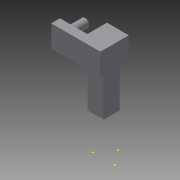
# Autodesk Inventor part: BearingEndCap
Saved by Autodesk Inventor 2015 (Build 190159000, 159)
## iProperties
Created: 2016-03-24
Part Number: BearingEndCap
Material: Generic
Document SubType Name: Modeling
Designer: Hatch
Density: 1 g/cm^3
Appearance: Default
Author: Hatch
Autodesk Inventor part; units mm, degrees
ref_plane "YZ Plane" through (0, 0, 0) normal (1, 0, 0) x (0, 1, 0)
ref_plane "XZ Plane" through (0, 0, 0) normal (0, 1, 0) x (-1, 0, 0)
ref_plane "XY Plane" through (0, 0, 0) normal (0, 0, 1) x (1, 0, 0)
sketch "Sketch1" plane through (0, 0, 0) normal (0, 1, 0) x (-1, 0, 0)
  line L0 (-7.25, 7.25) -> (7.25, 7.25)
  line L1 (7.25, 7.25) -> (7.25, -7.25)
  line L2 (7.25, -7.25) -> (-7.25, -7.25)
  line L3 (-7.25, -7.25) -> (-7.25, 7.25)
  line L4 (-7.25, 7.25) -> (7.25, -7.25) construction
  line L5 (7.25, 7.25) -> (-7.25, -7.25) construction
  point P0 (0, 0)
  dimension "d0" = 14.5
  dimension "d1" = 14.5
  constraints: 12 end point, 2 midpoint, 2 parallel, 1 horizontal, 1 perpendicular
  measures "d0" distance of L1.end L2.end
  measures "d1" distance of L0.end L1.end
extrude "Extrusion1" add sketch "Sketch1" along normal blind 76.2
sketch "Sketch2" plane through (0, 76.2, 0) normal (0, 1, 0) x (1, 0, 0)
  line L0 (10, -10) -> (-10, -10)
  line L1 (-10, -10) -> (-10, 10)
  line L2 (-10, 10) -> (10, 10)
  line L3 (10, 10) -> (10, -10)
  line L4 (10, -10) -> (-10, 10) construction
  line L5 (-10, -10) -> (10, 10) construction
  point P0 (0, 0)
  dimension "d4" = 20
  dimension "d5" = 20
  constraints: 12 end point, 2 midpoint, 2 parallel, 1 horizontal, 1 perpendicular
  measures "d4" distance of L1.end L2.end
  measures "d5" distance of L0.end L1.end
extrude "Extrusion2" add sketch "Sketch2" along normal blind 5
sketch "Sketch3" plane through (0, 81.2, 0) normal (0, 1, 0) x (1, 0, 0)
  line L0 (7.5, -7.5) -> (-7.5, -7.5)
  line L1 (-7.5, -7.5) -> (-7.5, 7.5)
  line L2 (-7.5, 7.5) -> (7.5, 7.5)
  line L3 (7.5, 7.5) -> (7.5, -7.5)
  line L4 (7.5, -7.5) -> (-7.5, 7.5) construction
  line L5 (-7.5, -7.5) -> (7.5, 7.5) construction
  line L6 (10, -10) -> (-10, -10)
  line L7 (-10, -10) -> (-10, 10)
  line L8 (-10, 10) -> (10, 10)
  line L9 (10, 10) -> (10, -10)
  line L10 (10, -10) -> (-10, 10) construction
  line L11 (-10, -10) -> (10, 10) construction
  point P0 (0, 0)
  dimension "d8" = 15
  dimension "d9" = 15
  constraints: 24 end point, 4 midpoint, 4 parallel, 2 horizontal, 2 perpendicular
  measures "d8" distance of L1.end L2.end
  measures "d9" distance of L0.end L1.end
extrude "Extrusion3" add sketch "Sketch3" along normal blind 76.2
sketch "Sketch4" plane through (10, 76.2, 10) normal (1, 0, 0) x (0, 0, -1)
  line L0 (20, 0) -> (20, 81.2) projected
  line L1 (15, 81.2) -> (15, 0)
  line L2 (0, 0) -> (20, 0) projected
  line L3 (15, 81.2) -> (13, 81.2)
  line L4 (17.5, 81.2) -> (2.5, 81.2) projected
  line L5 (13, 81.2) -> (13, 0)
  line L6 (13, 0) -> (15, 0)
  line L7 (20, 81.2) -> (0, 81.2) projected
  point P0 (10, -76.2)
  dimension "d12" = 2
  constraints: 8 end point, 3 point on line, 1 parallel, 1 perpendicular, 1 vertical
  measures "d12" distance of L1.start L3.end
extrude "Extrusion4" add sketch "Sketch4" along normal blind 10 contours L2 L5 L3 L1
sketch "Sketch5" plane through (10, 76.2, -3) normal (0, 0, 1) x (1, 0, 0)
  line L0 (0, 81.2) -> (10, 81.2) projected
  line L1 (10, 81.2) -> (8, 81.2)
  line L2 (8, 81.2) -> (8, 0)
  line L3 (8, 0) -> (10, 0)
  line L4 (10, 0) -> (10, 81.2)
  point P0 (-10, -76.2)
  dimension "d15" = 2
  constraints: 8 end point, 2 parallel, 1 perpendicular, 1 point on line
  measures "d15" distance of L0.end L1.end
extrude "Extrusion5" add sketch "Sketch5" along normal blind 8
sketch "Sketch6" plane through (20, 76.2, 10) normal (1, 0, 0) x (0, 0, -1)
  line L0 (5, 81.2) -> (3, 81.2)
  line L1 (3, 81.2) -> (3, 0)
  line L2 (3, 0) -> (5, 0)
  line L3 (5, 0) -> (5, 81.2)
  point P0 (10, -76.2)
  dimension "d18" = 2
  constraints: 8 end point, 2 parallel, 1 horizontal, 1 perpendicular
  measures "d18" distance of L0.start L0.end
extrude "Extrusion6" add sketch "Sketch6" against normal blind 4
sketch "Sketch7" plane through (0, 76.2, 0) normal (0, -1, 0) x (1, 0, 0)
  line L0 (10, -5) -> (20, -5)
  line L1 (20, -5) -> (20, 7)
  line L2 (20, 7) -> (10, 7)
  line L3 (10, 7) -> (10, -5)
  point P0 (0, 0)
  constraints: 8 end point, 2 parallel, 1 horizontal, 1 perpendicular
extrude "Extrusion7" cut sketch "Sketch7" against normal through all
sketch "Sketch8" plane through (7.25, 0, -7.25) normal (0, 0, -1) x (-1, 0, 0)
  line L0 (0, 0) -> (0, 76.2)
  line L1 (0, 0) -> (0, 76.2) projected
  line L2 (0, 38.1) -> (14.5, 38.1)
  line L3 (14.5, 38.1) -> (14.5, 0)
  line L4 (14.5, 0) -> (0, 0)
  line L5 (0, 0) -> (0, 38.1)
  point P0 (7.25, 0)
  constraints: 10 end point, 3 equal length, 1 horizontal, 1 midpoint, 1 perpendicular
extrude "Extrusion8" cut sketch "Sketch8" against normal through all
sketch "Sketch9" plane through (10, 76.2, -10) normal (0, 0, -1) x (-1, 0, 0)
  line L0 (0, 0) -> (0, 20)
  line L1 (0, 0) -> (0, 81.2) projected
  line L2 (0, 20) -> (20, 20)
  line L3 (20, 20) -> (20, 81.2)
  line L4 (20, 81.2) -> (0, 81.2)
  line L5 (0, 81.2) -> (0, 20)
  point P0 (10, -76.2)
  dimension "d25" = 20
  constraints: 10 end point, 2 parallel, 1 horizontal, 1 perpendicular, 1 point on line
  measures "d25" distance of L0.start L0.end
extrude "Extrusion9" cut sketch "Sketch9" against normal through all
sketch "Sketch10" plane through (-10, 96.2, -10) normal (0, 1, 0) x (1, 0, 0)
  line L0 (17.5, -2.5) -> (2.5, -2.5)
  line L1 (2.5, -2.5) -> (2.5, -17.5)
  line L2 (2.5, -17.5) -> (17.5, -17.5)
  line L3 (17.5, -17.5) -> (17.5, -2.5)
  point P0 (10, -10)
  constraints: 8 end point, 2 parallel, 1 horizontal, 1 perpendicular
extrude "Extrusion10" add sketch "Sketch10" against normal blind 15
sketch "Sketch11" plane through (10, 76.2, 10) normal (1, 0, 0) x (0, 0, -1)
  point P0 (10, -76.2)
sketch "Sketch12" plane through (-10, 76.2, -10) normal (-1, 0, 0) x (0, 0, 1)
  line L0 (0, 0) -> (0, 20) projected
  line L1 (20, 0) -> (20, 20) projected
  line L2 (20, 10) -> (15, 10)
  line L3 (0, 10) -> (5, 10)
  line L4 (20, 20) -> (23, 20)
  line L5 (23, 20) -> (23, 0)
  line L6 (23, 0) -> (20, 0)
  line L7 (20, 0) -> (20, 20)
  line L8 (0, 20) -> (-3, 20)
  line L9 (-3, 20) -> (-3, 0)
  line L10 (-3, 0) -> (0, 0)
  line L11 (0, 0) -> (0, 20)
  point P0 (10, -76.2)
  dimension "d30" = 5
  dimension "d31" = 5
  dimension "d32" = 3
  dimension "d33" = 3
  constraints: 20 end point, 4 horizontal, 4 parallel, 2 midpoint, 2 perpendicular, 1 point on line
  measures "d30" distance of L2.start L2.end
  measures "d31" distance of L3.start L3.end
  measures "d32" distance of L5.end L6.end
  measures "d33" distance of L10.end L9.end
extrude "Extrusion11" add sketch "Sketch12" against normal blind 20
sketch "Sketch13" plane through (-10, 76.2, -13) normal (-1, 0, 0) x (0, 0, 1)
  line L0 (20.25, 0) -> (5.75, 0) projected
  line L1 (0, 20) -> (8, 20)
  line L2 (8, 20) -> (8, 0)
  line L3 (8, 0) -> (0, 0)
  line L4 (0, 0) -> (0, 20)
  line L5 (26, 20) -> (18, 20)
  line L6 (18, 20) -> (18, 0)
  line L7 (18, 0) -> (26, 0)
  line L8 (26, 0) -> (26, 20)
  point P0 (13, -76.2)
  dimension "d36" = 8
  dimension "d37" = 8
  constraints: 16 end point, 4 parallel, 2 horizontal, 2 perpendicular, 2 point on line
  measures "d36" distance of L2.end L3.end
  measures "d37" distance of L7.end L6.end
extrude "Extrusion12" add sketch "Sketch13" along normal blind 25 contours L0 L6 L5 L8 L7
sketch "Sketch14" plane through (-10, 76.2, 5) normal (0, 0, -1) x (-1, 0, 0)
  line L0 (0, 20) -> (0, 0) projected
  line L1 (0, 10) -> (20, 10)
  circle A0 centre (20, 10) radius 3.75
  point P0 (-10, -76.2)
  dimension "d40" = 20
  dimension "d41" = 7.5
  constraints: 2 end point, 1 centre point, 1 coincident, 1 horizontal, 1 midpoint
  measures "d40" distance of L1.start L1.end
  measures "d41" diameter of A0
sketch "Sketch15" plane through (-10, 76.2, -13) normal (-1, 0, 0) x (0, 0, 1)
  point P0 (13, -76.2)
extrude "Extrusion13" add sketch "Sketch14" along normal blind 18
sketch "Sketch16" plane through (-10, 76.2, -13) normal (0, 0, -1) x (-1, 0, 0)
  point P0 (-10, -76.2)
body "Solid1"
